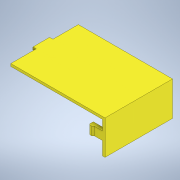
# Autodesk Inventor part: top
Saved by Autodesk Inventor 2022.2 (Build 262287000, 287)
## iProperties
Created: 2021-12-01
Part Number: top
Material: Generic
Document SubType Name: Modeling
Designer: samlo
Density: 1 g/cm^3
Appearance: Canary
Author: samlo
Autodesk Inventor part; units mm, degrees
ref_plane "YZ Plane" through (0, 0, 0) normal (1, 0, 0) x (0, 1, 0)
ref_plane "XZ Plane" through (0, 0, 0) normal (0, 1, 0) x (-1, 0, 0)
ref_plane "XY Plane" through (0, 0, 0) normal (0, 0, 1) x (1, 0, 0)
sketch "Sketch5" plane through (0, 0, 0) normal (0, 0, 1) x (1, 0, 0)
  line L0 (0, 0) -> (3, 0)
  line L1 (3, 0) -> (3, 41)
  line L2 (3, 41) -> (-110, 41)
  line L3 (-110, 41) -> (-110, 38)
  line L4 (-110, 38) -> (0, 38)
  line L5 (0, 38) -> (0, 0)
  dimension "d32" = 3
  dimension "d33" = 3
  dimension "d34" = 110
  dimension "d35" = 41
  constraints: 12 end point, 4 perpendicular, 1 horizontal
  measures "d32" distance of L0.start L0.end
  measures "d33" distance of L2.end L3.end
  measures "d34" distance of L3.end L4.end
  measures "d35" distance of L0.end L1.end
extrude "Extrusion4" add sketch "Sketch5" along normal blind 81
sketch "Sketch6" plane through (-110, 38, 0) normal (-1, 0, 0) x (0, 0, 1)
  line L0 (0, 0) -> (81, 0) projected
  line L1 (0, 3) -> (81, 3) projected
  line L2 (30.5, 0) -> (50.5, 0)
  line L3 (50.5, 0) -> (50.5, 3)
  line L4 (50.5, 3) -> (30.5, 3)
  line L5 (30.5, 3) -> (30.5, 0)
  point P0 (0, -38)
  point P1 (30.5, 3)
  dimension "d38" = 20
  dimension "d39" = 30.5
  constraints: 8 end point, 2 parallel, 2 point on line, 1 horizontal, 1 perpendicular
  measures "d38" distance of L2.start L2.end
  measures "d39" distance of L0.end L2.end
extrude "Extrusion5" add sketch "Sketch6" along normal blind 4
sketch "Sketch11" plane through (0, 0, 0) normal (-1, 0, 0) x (0, 0, 1)
  line L0 (81, 0) -> (81, 41) projected
  line L1 (81, 26) -> (77, 26)
  line L2 (77, 26) -> (77, 16)
  line L3 (77, 16) -> (81, 16)
  line L4 (81, 16) -> (81, 26)
  point P0 (0, 0)
  dimension "d67" = 4
  dimension "d68" = 10
  dimension "d69" = 16
  constraints: 8 end point, 2 parallel, 1 horizontal, 1 perpendicular, 1 point on line
  measures "d67" distance of L1.end L1.start
  measures "d68" distance of L1.end L2.end
  measures "d69" distance of L0.start L3.end
extrude "Extrusion6" add sketch "Sketch11" along normal blind 15
sketch "Sketch12" plane through (0, 0, 81) normal (0, 0, 1) x (1, 0, 0)
  line L0 (0, 16) -> (-15, 16) projected
  line L1 (-15, 26) -> (-10, 26)
  line L2 (-10, 26) -> (-10, 16)
  line L3 (-10, 16) -> (-15, 16)
  line L4 (-15, 16) -> (-15, 26)
  point P0 (0, 0)
  dimension "d72" = 10
  constraints: 8 end point, 2 parallel, 1 horizontal, 1 perpendicular, 1 point on line
  measures "d72" distance of L0.start L2.end
extrude "Extrusion7" add sketch "Sketch12" along normal blind 1.5
sketch "Sketch13" plane through (0, 16, 77) normal (0, -1, 0) x (1, 0, 0)
  line L0 (-110, 4) -> (0, 4) projected
  line L1 (-15.0054, 4) -> (-13.7468, 5.5)
  line L2 (-10, 5.5) -> (-15, 5.5) projected
  line L3 (-15.0054, 5.5) -> (-15.0054, 4)
  line L4 (-15, 0) -> (-15, 5.5) projected
  line L5 (0, 4) -> (-10, 4) projected
  line L6 (-15.0054, 5.5) -> (-13.7468, 5.5)
  point P0 (0, -77)
  dimension "d75" = 50
  constraints: 6 end point, 2 point on line, 1 collinear, 1 parallel
  measures "d75" angle of L1 L2
extrude "Extrusion8" cut sketch "Sketch13" against normal up to surface (10 mm away) contours L3 L6 L4 L1 | L4 L2 L1
sketch "Sketch14" plane through (0, 16, 77) normal (0, -1, 0) x (1, 0, 0)
  line L0 (0, 4) -> (-10, 4) projected
  line L1 (-10, 4) -> (-11.2586, 5.5)
  line L2 (-13.7468, 5.5) -> (-10, 5.5) projected
  line L3 (-10, 4) -> (-10, 5.5) projected
  line L4 (-10, 5.5) -> (-10, 4)
  point P0 (0, -77)
  dimension "d78" = 50
  constraints: 4 end point, 1 point on line, 1 vertical
  measures "d78" angle of L1 L2
extrude "Extrusion9" cut sketch "Sketch14" against normal up to surface (10 mm away)
ref_plane "Work Plane3" through (0, 0, 40.5) normal (0, 0, 1) x (1, 0, 0)
mirror "Mirror4" about plane through (0, 0, 40.5) normal (0, 0, 1) of "Extrusion6"
mirror "Mirror5" about plane through (0, 0, 40.5) normal (0, 0, 1) of "Extrusion7"
mirror "Mirror6" about plane through (0, 0, 40.5) normal (0, 0, 1) of "Extrusion8"
mirror "Mirror7" about plane through (0, 0, 40.5) normal (0, 0, 1) of "Extrusion9"
body "Solid2"
